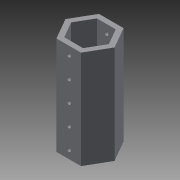
# Autodesk Inventor part: agujereador
Saved by Autodesk Inventor 2015 SP1 (Build 190203100, 203)
## iProperties
Created: 2015-06-22
Part Number: agujereador
Material: Genérico
Document SubType Name: Modeling
Designer: Javier
Density: 1 g/cm^3
Appearance: Valor por defecto
Author: Javier
Autodesk Inventor part; units mm, degrees
ref_plane "YZ Plane" through (0, 0, 0) normal (1, 0, 0) x (0, 1, 0)
ref_plane "XZ Plane" through (0, 0, 0) normal (0, 1, 0) x (-1, 0, 0)
ref_plane "XY Plane" through (0, 0, 0) normal (0, 0, 1) x (1, 0, 0)
sketch "Boceto1" plane through (0, 0, 0) normal (0, 0, 1) x (1, 0, 0)
  line L0 (4.6, 0) -> (2.3, -3.9837)
  line L1 (2.3, -3.9837) -> (-2.3, -3.9837)
  line L2 (-2.3, -3.9837) -> (-4.6, 0)
  line L3 (-4.6, 0) -> (-2.3, 3.9837)
  line L4 (-2.3, 3.9837) -> (2.3, 3.9837)
  line L5 (2.3, 3.9837) -> (4.6, 0)
  line L6 (6, 0) -> (3, -5.1962)
  line L7 (3, -5.1962) -> (-3, -5.1962)
  line L8 (-3, -5.1962) -> (-6, 0)
  line L9 (-6, 0) -> (-3, 5.1962)
  line L10 (-3, 5.1962) -> (3, 5.1962)
  line L11 (3, 5.1962) -> (6, 0)
  point P0 (0, 0)
  point P1 (0, 0)
  point P2 (0, 0)
  dimension "d0" = 9.2
  dimension "d1" = 12
  constraints: 24 end point, 2 coincident, 26 other
  measures "d0" distance of L0.start L2.end
  measures "d1" distance of L6.start L8.end
extrude "Extrusión1" add sketch "Boceto1" along normal blind 24
sketch "Boceto2" plane through (-3, 5.1962, 0) normal (0, 1, 0) x (1, 0, 0)
  line L0 (0, 0) -> (6, 0) projected
  line L1 (0, 0) -> (0, -24) projected
  line L2 (6, -24) -> (0, -24) projected
  line L3 (6, 0) -> (6, -24) projected
  line L4 (3, -24) -> (3, -22)
  line L5 (3, -22) -> (3, -17)
  line L6 (3, -17) -> (3, -12)
  line L7 (3, -12) -> (3, -7)
  line L8 (3, -7) -> (3, -2)
  line L9 (3, -2) -> (3, 0)
  circle A0 centre (3, -22) radius 0.5
  circle A1 centre (3, -17) radius 0.5
  circle A2 centre (3, -12) radius 0.5
  circle A3 centre (3, -7) radius 0.5
  circle A4 centre (3, -2) radius 0.5
  dimension "d4" = 2
  dimension "d5" = 5
  dimension "d6" = 5
  dimension "d7" = 5
  dimension "d8" = 5
  dimension "d9" = 1
  dimension "d10" = 1
  dimension "d11" = 1
  dimension "d12" = 1
  dimension "d13" = 1
  constraints: 12 end point, 5 centre point, 5 coincident, 4 point on line, 1 collinear, 1 midpoint, 1 vertical
  measures "d4" distance of L4.start L4.end
  measures "d5" distance of L4.end L5.end
  measures "d6" distance of L5.end L6.end
  measures "d7" distance of L6.end L7.end
  measures "d8" distance of L7.end L8.end
  measures "d9" diameter of A0
  measures "d10" diameter of A1
  measures "d11" diameter of A2
  measures "d12" diameter of A3
  measures "d13" diameter of A4
extrude "Extrusión2" cut sketch "Boceto2" against normal blind 24 contours A4 L8 L9 | L9 L8 A4 | A0 L5 L4 | L4 L5 A0 | A3 L7 L8 | L8 L7 A3 | A1 L6 L5 | L5 L6 A1 | A2 L6 L7 | L7 L6 A2
